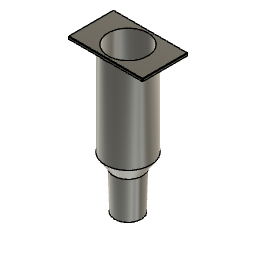
dpv2_syringe (Autodesk Fusion 360 design; units mm, degrees)
Autodesk Fusion 360 part; units mm, degrees
sketch "スケッチ3" plane through (0, 0, 0) normal (0, 1, 0) x (1, 0, 0)
  line L0 (5.65, 0) -> (6.2, -20.4286)
  line L1 (6.2, -20.4286) -> (10.7, -27.7598)
  line L2 (10.7, -27.7598) -> (10.7, -77.7598)
  line L3 (10.7, -77.7598) -> (12.2, -77.7598)
  line L4 (12.2, -77.7598) -> (12.2, -27.7598)
  line L5 (12.2, -27.7598) -> (7.7, -20.4286)
  line L6 (7.7, -20.4286) -> (7.15, 0)
  line L7 (7.15, 0) -> (5.65, 0)
  line L8 (1.75, 0) -> (22.5, 0)
  line L9 (6.2, -20.4286) -> (7.7, -20.4286) construction
  line L10 (12.2, -27.7598) -> (10.7, -27.7598) construction
  point P0 (7.55, -14.8571)
  point P1 (7.2, -1.8571)
  dimension "d46" = 7.55
  dimension "d47" = 7.2
  dimension "d48" = 13
  dimension "d49" = 10.7
  dimension "d51" = 1.5
  dimension "d52" = 50
  dimension "d54" = 150
  dimension "d56" = 7.15
  dimension "d57" = 7.7
  constraint vertical L2
  constraint perpendicular L2 L3
  constraint perpendicular L3 L4
  constraint parallel L0 L6
  constraint collinear L7 L8
  constraint coincident L6 P0
  constraint coincident L6 P1
  constraint parallel L8 L9
  constraint parallel L1 L5
  constraint parallel L8 L10
  measures "d46" horizontal distance of origin P0
  measures "d47" horizontal distance of origin P1
  measures "d48" vertical distance of P0 P1
  measures "d49" distance of origin L2
  measures "d51" distance of L0.start L6.end
  measures "d52" distance of L3.end L4.end
  measures "d54" angle of L5 L6
  measures "d56" distance of origin L6.end
  measures "d57" horizontal distance of origin L5.end
revolve "回転2" add sketch "スケッチ3" angle 360 about axis through (0, 0, 1.75) along (0, 0, 1)
sketch "スケッチ4" plane through (0, 0, 77.7598) normal (0, 0, 1) x (-1, 0, 0)
  circle A0 centre (0, 0) radius 12.2
  circle A1 centre (0, 0) radius 10.7
  line L0 (20, -12.2) -> (-20, -12.2)
  line L1 (-20, -12.2) -> (-20, 12.2)
  line L2 (-20, 12.2) -> (20, 12.2)
  line L3 (20, 12.2) -> (20, -12.2)
  line L4 (0, -1.75) -> (0, -22.5)
  dimension "d58" = 40
  constraint horizontal L0
  constraint vertical L1
  constraint horizontal L2
  constraint vertical L3
  constraint tangent A0 L0
  constraint tangent A0 L2
  constraint symmetric L1 L3 L4
  measures "d58" distance of L0.start L0.end
extrude "押し出し1" add sketch "スケッチ4" against normal blind 1.5 contours A0 L0 L2 L3 | A0 L0 L1 L2
fillet "フィレット1" radius 0.25 14 edges at (0, 12.2, 77.7598) (20, 0, 77.7598) (0, -12.2, 77.7598) (-20, 0, 77.7598) (20, -12.2, 77.0098) (-20, -12.2, 77.0098) (-10, -12.2, 76.2598) (10, -12.2, 76.2598) (20, 0, 76.2598) (20, 12.2, 77.0098) (10, 12.2, 76.2598) (-10, 12.2, 76.2598) (-20, 12.2, 77.0098) (-20, 0, 76.2598)
